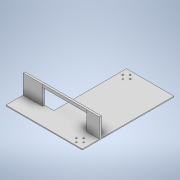
# Autodesk Inventor part: Plate
Saved by Autodesk Inventor 2020 (Build 240168000, 168)
## iProperties
Created: 2020-11-25
Part Number: Plate
Material: Generic
Document SubType Name: Modeling
Designer: tdmp4
Density: 1 g/cm^3
Appearance: Default
Author: tdmp4
Autodesk Inventor part; units mm, degrees
ref_plane "YZ Plane" through (0, 0, 0) normal (1, 0, 0) x (0, 1, 0)
ref_plane "XZ Plane" through (0, 0, 0) normal (0, 1, 0) x (-1, 0, 0)
ref_plane "XY Plane" through (0, 0, 0) normal (0, 0, 1) x (1, 0, 0)
sketch "Sketch1" plane through (0, 0, 0) normal (0, 1, 0) x (-1, 0, 0)
  line L0 (0, 0) -> (177.8, 0)
  line L1 (177.8, 0) -> (177.8, -243.078)
  line L2 (177.8, -243.078) -> (0, -243.078)
  line L3 (0, -243.078) -> (0, 0)
  dimension "d0" = 243.078
  dimension "d1" = 177.8
  constraints: 8 end point, 2 parallel, 1 horizontal, 1 perpendicular
  measures "d0" distance of L0.end L1.end
  measures "d1" distance of L1.end L2.end
extrude "Extrusion1" add sketch "Sketch1" along normal blind 2.286
sketch "Sketch2" plane through (0, 2.286, 0) normal (0, 1, 0) x (1, 0, 0)
  circle A0 centre (-75.024, 26.7891) radius 1.905
  circle A1 centre (-65.245, 17.0101) radius 1.905
  circle A2 centre (-75.024, 7.2311) radius 1.905
  circle A3 centre (-84.803, 17.0101) radius 1.905
  dimension "d7" = 3.81
  dimension "d8" = 3.81
  dimension "d9" = 3.81
  dimension "d10" = 3.81
  constraints: 4 centre point
  measures "d7" diameter of A0
  measures "d8" diameter of A1
  measures "d9" diameter of A2
  measures "d10" diameter of A3
extrude "Extrusion2" cut sketch "Sketch2" against normal blind 5.461
sketch "Sketch4" plane through (0, 2.286, 0) normal (0, 1, 0) x (1, 0, 0)
  line L0 (0, 0) -> (-177.8, 0)
  line L1 (-177.8, 0) -> (-177.8, 50.8)
  line L2 (-177.8, 50.8) -> (0, 50.8)
  line L3 (0, 50.8) -> (0, 45.5143)
  line L4 (0, 0) -> (0, 243.078) projected
  line L5 (0, 45.5143) -> (-177.8, 45.5143)
  line L6 (-85.237, 50.8) -> (-85.237, 45.5143)
  point P0 (0, 188.468)
  dimension "d16" = 50.8
  constraints: 12 end point, 4 point on line, 2 perpendicular, 1 horizontal, 1 parallel
  measures "d16" distance of L2.end L0.start
extrude "Extrusion4" add sketch "Sketch4" along normal blind 50.8 contours L5 L6 L2 L3
sketch "Sketch6" plane through (-177.8, 0, -243.078) normal (-1, 0, 0) x (0, 0, 1)
  line L0 (243.078, 0) -> (0, 0) projected
  line L1 (0, 2.286) -> (243.078, 2.286) projected
  line L2 (243.078, 0) -> (192.4335, 0)
  line L3 (192.4335, 0) -> (192.4335, 2.286)
  line L4 (192.4335, 2.286) -> (243.078, 2.286)
  line L5 (243.078, 2.286) -> (243.078, 0)
  point P0 (3.81, 2.286)
  point P1 (243.078, 2.286)
  point P2 (192.4335, 0)
  dimension "d28" = 243.078
  constraints: 8 end point, 2 parallel, 1 horizontal, 1 perpendicular, 1 point on line
  measures "d28" distance of L0.start L0.end
extrude "Extrusion6" add sketch "Sketch6" along normal blind 76.2
sketch "Sketch7" plane through (0, 2.286, 0) normal (0, 1, 0) x (1, 0, 0)
  line L0 (-177.8, 50.6445) -> (-254, 50.6445) projected
  line L1 (-254, 50.6445) -> (-203.1257, 50.6445)
  line L2 (-203.1257, 50.6445) -> (-203.1257, 45.5645)
  line L3 (-203.1257, 45.5645) -> (-254, 45.5645)
  line L4 (-254, 45.5645) -> (-254, 50.6445)
  point P0 (0, 0)
  dimension "d31" = 5.08
  constraints: 8 end point, 2 parallel, 1 horizontal, 1 perpendicular
  measures "d31" distance of L3.end L0.end
extrude "Extrusion7" add sketch "Sketch7" along normal blind 50.8
sketch "Sketch8" plane through (0, 2.286, -50.8) normal (0, 0, -1) x (-1, 0, 0)
  line L0 (0, 50.8) -> (85.237, 50.8) projected
  line L1 (203.1257, 0) -> (203.1257, 50.8) projected
  line L2 (85.237, 50.8) -> (203.1257, 50.8)
  line L3 (203.1257, 50.8) -> (203.1257, 43.18)
  line L4 (203.1257, 43.18) -> (85.237, 43.18)
  line L5 (85.237, 43.18) -> (85.237, 50.8)
  point P0 (0, -2.286)
  dimension "d34" = 50.8
  dimension "d35" = 7.62
  constraints: 8 end point, 2 parallel, 1 horizontal, 1 perpendicular, 1 point on line
  measures "d34" distance of L1.start L1.end
  measures "d35" distance of L4.end L0.end
extrude "Extrusion8" add sketch "Sketch8" against normal blind 5.08
sketch "Sketch10" plane through (0, 53.086, 0) normal (0, 1, 0) x (1, 0, 0)
  line L0 (0, 0) -> (-254, 0) projected
  line L1 (0, 188.468) -> (-177.8, 188.468) projected
  line L2 (-51.904, 0) -> (0, 0)
  line L3 (0, 0) -> (0, 188.468)
  line L4 (0, 188.468) -> (-51.904, 188.468)
  line L5 (-51.904, 188.468) -> (-51.904, 0)
  line L6 (0, 243.078) -> (-177.8, 243.078) projected
  line L7 (-51.904, 188.468) -> (0, 188.468)
  line L8 (0, 188.468) -> (0, 243.078)
  line L9 (0, 243.078) -> (-51.904, 243.078)
  line L10 (-51.904, 243.078) -> (-51.904, 188.468)
  constraints: 16 end point, 4 parallel, 2 horizontal, 2 perpendicular, 1 point on line
extrude "Extrusion9" cut sketch "Sketch10" against normal blind 87.3125
sketch "Sketch11" plane through (0, 2.286, 0) normal (0, 1, 0) x (1, 0, 0)
  line L0 (-177.8, 243.078) -> (-177.8, 50.6445) projected
  line L1 (-177.8, 243.078) -> (-139.7, 243.078)
  line L2 (-139.7, 243.078) -> (-139.7, 204.978)
  line L3 (-139.7, 204.978) -> (-177.8, 204.978)
  line L4 (-177.8, 204.978) -> (-177.8, 243.078)
  circle A0 centre (-158.75, 224.028) radius 9.779
  circle A1 centre (-168.529, 224.028) radius 1.905
  circle A2 centre (-158.75, 233.807) radius 1.905
  circle A3 centre (-158.75, 214.249) radius 1.4605
  circle A4 centre (-148.971, 224.028) radius 1.905
  point P0 (0, 0)
  dimension "d40" = 38.1
  dimension "d41" = 38.1
  dimension "d42" = 19.558
  dimension "d43" = 3.81
  dimension "d44" = 3.81
  dimension "d45" = 2.921
  dimension "d46" = 3.81
  constraints: 8 end point, 5 centre point, 4 point on circle, 2 parallel, 1 horizontal, 1 perpendicular
  measures "d40" distance of L2.end L3.end
  measures "d41" distance of L1.end L2.end
  measures "d42" diameter of A0
  measures "d43" diameter of A1
  measures "d44" diameter of A2
  measures "d45" diameter of A3
  measures "d46" diameter of A4
extrude "Extrusion10" cut sketch "Sketch11" against normal blind 25.4 contours A0 A4 | A0 A4 | A2 A0 | A0 A2 | A3 A0 | A0 A3 | A1 A0 | A0 A1
body "Solid1"
